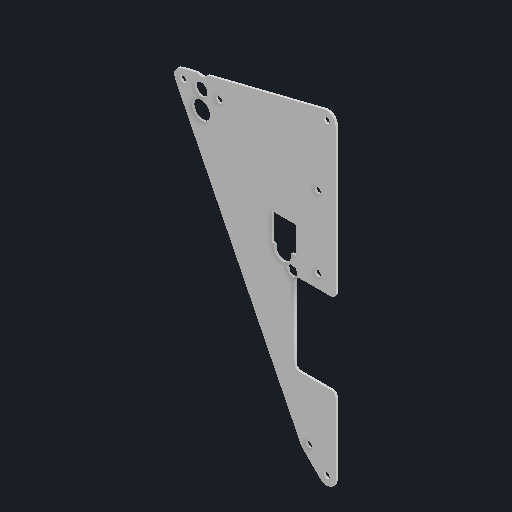
# Autodesk Inventor part: outer-tower-support-proto
Saved by Autodesk Inventor 2023 (Build 270158000, 158)
## iProperties
Created: 2023-03-21
Part Number: outer-tower-support-proto
Material: Generic
Document SubType Name: Modeling
Designer: Liam
Density: 1 g/cm^3
Appearance: Default
Author: Liam
Autodesk Inventor part; units mm, degrees
ref_plane "YZ Plane" through (0, 0, 0) normal (1, 0, 0) x (0, 1, 0)
ref_plane "XZ Plane" through (0, 0, 0) normal (0, 1, 0) x (-1, 0, 0)
ref_plane "XY Plane" through (0, 0, 0) normal (0, 0, 1) x (1, 0, 0)
sketch "Sketch1" plane through (0, 0, 0) normal (0, 0, 1) x (1, 0, 0)
  circle A0 centre (-71.4375, -30.1625) radius 6.35
  line L0 (12.9724, -214.0401) -> (0.2724, -201.3401)
  line L1 (-0.9271, -199.6696) -> (-89.8271, -20.2821)
  line L2 (23.8125, 7.9375) -> (23.8125, -44.45)
  arc A1 (12.9724, -214.0401) -> (23.8125, -209.55) centre (17.4625, -209.55) ccw
  arc A2 (-0.9271, -199.6696) -> (0.2724, -201.3401) centre (4.7625, -196.85) ccw
  arc A3 (-85.6776, -11.3021) -> (-89.8271, -20.2821) centre (-84.1375, -17.4625) ccw
  arc A4 (23.8125, 7.9375) -> (15.9224, 14.0979) centre (17.4625, 7.9375) ccw
  circle A5 centre (-71.4375, -17.4625) radius 2.1844
  line L3 (-85.6776, -11.3021) -> (-75.211, -8.6854)
  line L4 (15.9224, 14.0979) -> (-66.2619, -6.4482)
  arc A6 (-73.1895, -8.8477) -> (-67.9692, -7.5426) centre (-71.4375, -4.7625) ccw
  arc A7 (-66.2619, -6.4482) -> (-67.9692, -7.5426) centre (-65.4918, -9.5284) ccw
  arc A8 (-73.1895, -8.8477) -> (-75.211, -8.6854) centre (-74.4409, -11.7656) ccw
  circle A9 centre (-71.4375, -17.4625) radius 4.445
  circle A10 centre (11.1125, -88.9) radius 2.2098
  line L5 (23.8125, -158.825) -> (23.8125, -209.55)
  line L6 (23.8125, -44.45) -> (23.8125, -95.175)
  circle A11 centre (17.4625, 7.9375) radius 2.1082
  circle A12 centre (-84.1375, -17.4625) radius 2.1082
  circle A13 centre (-58.7375, -17.4625) radius 2.1844 projected
  circle A14 centre (11.1125, -38.1) radius 2.1844 projected
  circle A15 centre (17.4625, -209.55) radius 2.1082
  circle A16 centre (4.7625, -196.85) radius 2.1082
  line L7 (-9.6199, -99.1398) -> (-10.6249, -95.4647) projected
  line L8 (-5.9347, -100.107) -> (-9.6199, -99.1398) projected
  line L9 (-3.2545, -97.3991) -> (-5.9347, -100.107) projected
  line L10 (-4.2595, -93.724) -> (-3.2545, -97.3991) projected
  line L11 (-7.9447, -92.7568) -> (-4.2595, -93.724) projected
  line L12 (-10.6249, -95.4647) -> (-7.9447, -92.7568) projected
  circle A17 centre (-13.7795, -88.1118) radius 2.0955 projected
  line L13 (-21.3274, -85.3813) -> (-21.3274, -67.4667)
  line L14 (-20.6924, -66.8317) -> (-4.8945, -66.8317)
  line L15 (-4.2595, -67.4667) -> (-4.2595, -85.3813)
  arc A18 (-19.4799, -86.7943) -> (-8.0791, -86.7943) centre (-13.7795, -88.1118) ccw
  line L16 (-7.4604, -86.0163) -> (-4.8945, -86.0163)
  line L17 (-20.0986, -86.0163) -> (-20.6924, -86.0163)
  arc A19 (-7.4604, -86.0163) -> (-8.0791, -86.7943) centre (-7.4604, -86.6513) ccw
  arc A20 (-19.4799, -86.7943) -> (-20.0986, -86.0163) centre (-20.0986, -86.6513) ccw
  arc A21 (-21.3274, -85.3813) -> (-20.6924, -86.0163) centre (-20.6924, -85.3813) ccw
  arc A22 (-4.8945, -86.0163) -> (-4.2595, -85.3813) centre (-4.8945, -85.3813) ccw
  arc A23 (-4.2595, -67.4667) -> (-4.8945, -66.8317) centre (-4.8945, -67.4667) ccw
  arc A24 (-20.6924, -66.8317) -> (-21.3274, -67.4667) centre (-20.6924, -67.4667) ccw
  line L18 (23.8125, -94.6995) -> (23.8125, -97.7374)
  line L19 (-1.7875, -98.35) -> (20.6375, -98.35)
  arc A25 (-1.7875, -98.35) -> (-5.3875, -101.95) centre (-1.7875, -101.95) ccw
  line L20 (-5.3875, -108.7656) -> (-5.3875, -101.95)
  line L21 (-5.3875, -152.05) -> (-5.3875, -108.7656)
  arc A26 (-5.3875, -152.05) -> (-1.7875, -155.65) centre (-1.7875, -152.05) ccw
  line L22 (20.6375, -155.65) -> (-1.7875, -155.65)
  arc A27 (23.8125, -158.825) -> (20.6375, -155.65) centre (20.6375, -158.825) ccw
  arc A28 (20.6375, -98.35) -> (23.8125, -95.175) centre (20.6375, -95.175) ccw
  point P0 (0, 0)
  point P1 (-74.0123, -8.3858)
  point P2 (-67.4605, -6.7478)
  point P3 (16.6133, -60.3277)
  point P4 (-19.242, -86.0163)
  point P5 (-8.317, -86.0163)
  dimension "d13" = 12.7
  dimension "d30" = 4.3688
  dimension "d32" = 3.175
  dimension "d33" = 8.89
  dimension "d34" = 4.4196
  dimension "d51" = 4.2164
  dimension "d52" = 4.2164
  dimension "d54" = 4.2164
  dimension "d55" = 4.2164
  dimension "d56" = 0.635
  dimension "d59" = 3.175
  constraints: 40 point on circle, 34 end point, 26 centre point, 20 tangent, 7 equal radius, 6 point on line, 5 coincident, 3 vertical, 1 horizontal, 1 parallel, 1 perpendicular, 5 other
  measures "d13" diameter of A0
  measures "d30" diameter of A5
  measures "d32" radius of A7
  measures "d33" diameter of A9
  measures "d34" diameter of A10
  measures "d51" diameter of A11
  measures "d52" diameter of A12
  measures "d54" diameter of A15
  measures "d55" diameter of A16
  measures "d56" radius of A19
  measures "d59" radius of A27
extrude "Extrusion6" add sketch "Sketch1" along normal blind 1.524 contours L0 A2 L1 A3 L3 A8 A6 A7 L4 A4 L2 L6 A28 L19 A25 L20 L21 A26 L22 A27 L5 A1
body "Solid6"
